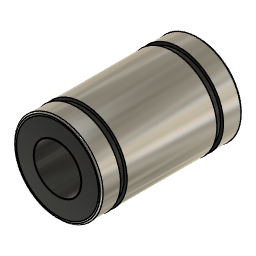
LM8UU (Autodesk Fusion 360 design; units mm, degrees)
Autodesk Fusion 360 part; units mm, degrees
sketch "front" plane through (0, 0, 0) normal (0, 1, 0) x (1, 0, 0) in component "LM8UU"
  circle A0 centre (0, 0) radius 4
  circle A1 centre (0, 0) radius 7
  circle A2 centre (0, 0) radius 7.5
  circle A3 centre (0, 0) radius 4.1
  dimension "d1" = 8
  dimension "d2" = 14
  dimension "d3" = 15
  dimension "d20" = 8.2
  constraint coincident A0.centre A1.centre
  constraint concentric A0 A1
  constraint concentric A1 A3
  measures "d1" diameter of A0
  measures "d2" diameter of A1
  measures "d3" diameter of A2
  measures "d20" diameter of A3
extrude "Extrude1" add sketch "front" along normal blind 3.25 contours A1 | A2 | A3 in component "LM8UU"
extrude "Extrude2" add sketch "front" along normal blind 1.1 from surface at 3.25 contours A1 | A3 in component "LM8UU"
extrude "Extrude3" add sketch "front" along normal blind 15.3 from surface at 4.35 contours A1 | A2 | A3 in component "LM8UU"
extrude "Extrude4" add sketch "front" along normal blind 1.1 from surface at 19.65 contours A1 | A3 in component "LM8UU"
extrude "Extrude5" add sketch "front" along normal blind 3.25 from surface at 20.75 contours A1 | A2 | A3 in component "LM8UU"
fillet "Fillet1" radius 0.25 2 edges at (-6.9925, 0, 2.7121) (-6.9925, 24, 2.7121) in component "LM8UU"
extrude "Extrude6" cut sketch "front" along normal blind 0.01 contours A1 in component "LM8UU"
extrude "Extrude7" cut sketch "front" along normal blind 0.01 from surface at 23.99 contours A1 in component "LM8UU"
component "LM8UU" placed x (1, 0, 0) y (0, 1, 0) z (0, 0, 1) at (0, 0, 0)
equation "d9 = 3.25 mm + 1.1 mm"
equation "d10 = 17.5 mm - 2.2 mm"
equation "d12 = 3.25 mm + 17.5 mm - 1.1 mm"
equation "d15 = 3.25 mm + 17.5 mm"
equation "d23 = 24 mm - 0.01 mm"
named bodies: "bearing"
